Autodesk Inventor part; units mm, degrees
(part 2 of 2)
  spline S114 degree 2 poles (-84.0515, 70.7348) (-84.2812, 70.7348) (-84.6789, 70.8583) (-84.8098, 70.9275) knots 0 0 0 1 2 2 2
  line L120 (-84.8098, 70.9275) -> (-84.8098, 71.3597)
  line L121 (-84.8098, 71.3597) -> (-84.79, 71.3597)
  spline S115 degree 2 poles (-84.79, 71.3597) (-84.7406, 71.3202) (-84.6072, 71.2263) (-84.4961, 71.1745) knots 0 0 0 1 2 2 2
  spline S116 degree 2 poles (-84.4961, 71.1745) (-84.3997, 71.1275) (-84.1626, 71.0584) (-84.0367, 71.0584) knots 0 0 0 1 2 2 2
  spline S117 degree 2 poles (-84.0367, 71.0584) (-83.9453, 71.0584) (-83.7353, 71.1004) (-83.6859, 71.1349) knots 0 0 0 1 2 2 2
  spline S118 degree 2 poles (-83.6859, 71.1349) (-83.6143, 71.1819) (-83.5501, 71.2881) (-83.5501, 71.3968) knots 0 0 0 1 2 2 2
  spline S119 degree 2 poles (-83.5501, 71.3968) (-83.5501, 71.5326) (-83.6983, 71.6734) (-83.8885, 71.7203) knots 0 0 0 1 2 2 2
  spline S120 degree 2 poles (-83.8885, 71.7203) (-83.9626, 71.7376) (-84.1997, 71.787) (-84.3009, 71.8142) knots 0 0 0 1 2 2 2
  spline S121 degree 2 poles (-84.3009, 71.8142) (-84.5628, 71.8908) (-84.7999, 72.2069) (-84.7999, 72.4317) knots 0 0 0 1 2 2 2
  spline S122 degree 2 poles (-84.7999, 72.4317) (-84.7999, 72.7429) (-84.3331, 73.1307) (-83.9477, 73.1307) knots 0 0 0 1 2 2 2
  spline S123 degree 2 poles (-83.9477, 73.1307) (-83.7575, 73.1307) (-83.3722, 73.0369) (-83.2413, 72.9652) knots 0 0 0 1 2 2 2
  line L122 (-83.2413, 72.9652) -> (-83.2413, 72.5527)
  line L123 (-83.2413, 72.5527) -> (-83.2611, 72.5527)
  spline S124 degree 2 poles (-83.2611, 72.5527) (-83.4093, 72.6713) (-83.7699, 72.8071) (-83.9551, 72.8071) knots 0 0 0 1 2 2 2
  spline S125 degree 2 poles (-83.9551, 72.8071) (-84.1453, 72.8071) (-84.4072, 72.6466) (-84.4072, 72.486) knots 0 0 0 1 2 2 2
  spline S126 degree 2 poles (-84.4072, 72.486) (-84.4072, 72.3403) (-84.2515, 72.1995) (-84.0786, 72.1551) knots 0 0 0 1 2 2 2
  spline S127 degree 2 poles (-84.0786, 72.1551) (-83.9947, 72.1328) (-83.7822, 72.0884) (-83.6662, 72.0612) knots 0 0 0 1 2 2 2
  spline S128 degree 2 poles (-83.6662, 72.0612) (-83.4142, 71.997) (-83.1573, 71.703) (-83.1573, 71.4486) knots 0 0 0 1 2 2 2
  spline S129 degree 2 poles (-83.1573, 71.4486) (-83.1573, 71.3004) (-83.2734, 71.0386) (-83.387, 70.9423) knots 0 0 0 1 2 2 2
  spline S130 degree 2 poles (-83.387, 70.9423) (-83.5081, 70.841) (-83.8168, 70.7348) (-84.0515, 70.7348) knots 0 0 0 1 2 2 2
  spline S131 degree 2 poles (-82.1076, 70.7447) (-82.4213, 70.7447) (-82.7745, 71.1028) (-82.7745, 71.4906) knots 0 0 0 1 2 2 2
  line L124 (-82.7745, 71.4906) -> (-82.7745, 72.7577)
  line L125 (-82.7745, 72.7577) -> (-83.0338, 72.7577)
  line L126 (-83.0338, 72.7577) -> (-83.0338, 73.0764)
  line L127 (-83.0338, 73.0764) -> (-82.7745, 73.0764)
  line L128 (-82.7745, 73.0764) -> (-82.7745, 73.7334)
  line L129 (-82.7745, 73.7334) -> (-82.3892, 73.7334)
  line L130 (-82.3892, 73.7334) -> (-82.3892, 73.0764)
  line L131 (-82.3892, 73.0764) -> (-81.6803, 73.0764)
  line L132 (-81.6803, 73.0764) -> (-81.6803, 72.7577)
  line L133 (-81.6803, 72.7577) -> (-82.3892, 72.7577)
  line L134 (-82.3892, 72.7577) -> (-82.3892, 71.6685)
  spline S132 degree 2 poles (-82.3892, 71.6685) (-82.3892, 71.4956) (-82.3768, 71.3054) (-82.3348, 71.2239) knots 0 0 0 1 2 2 2
  spline S133 degree 2 poles (-82.3348, 71.2239) (-82.3002, 71.1522) (-82.1446, 71.0806) (-82.0112, 71.0806) knots 0 0 0 1 2 2 2
  spline S134 degree 2 poles (-82.0112, 71.0806) (-81.9174, 71.0806) (-81.742, 71.1374) (-81.7025, 71.1547) knots 0 0 0 1 2 2 2
  line L135 (-81.7025, 71.1547) -> (-81.6803, 71.1547)
  line L136 (-81.6803, 71.1547) -> (-81.6803, 70.8089)
  spline S135 degree 2 poles (-81.6803, 70.8089) (-81.7889, 70.7793) (-82.0112, 70.7447) (-82.1076, 70.7447) knots 0 0 0 1 2 2 2
  line L137 (-79.3461, 70.7891) -> (-79.3461, 73.4765)
  line L138 (-79.3461, 73.4765) -> (-80.3687, 73.4765)
  line L139 (-80.3687, 73.4765) -> (-80.3687, 73.8371)
  line L140 (-80.3687, 73.8371) -> (-77.9184, 73.8371)
  line L141 (-77.9184, 73.8371) -> (-77.9184, 73.4765)
  line L142 (-77.9184, 73.4765) -> (-78.941, 73.4765)
  line L143 (-78.941, 73.4765) -> (-78.941, 70.7891)
  line L144 (-78.941, 70.7891) -> (-79.3461, 70.7891)
  line L145 (-75.8436, 73.0764) -> (-77.0737, 69.9469)
  line L146 (-77.0737, 69.9469) -> (-77.4862, 69.9469)
  line L147 (-77.4862, 69.9469) -> (-77.0762, 70.9003)
  line L148 (-77.0762, 70.9003) -> (-77.9061, 73.0764)
  line L149 (-77.9061, 73.0764) -> (-77.4911, 73.0764)
  line L150 (-77.4911, 73.0764) -> (-76.8662, 71.3819)
  line L151 (-76.8662, 71.3819) -> (-76.2438, 73.0764)
  line L152 (-76.2438, 73.0764) -> (-75.8436, 73.0764)
  spline S136 degree 2 poles (-73.6354, 71.9945) (-73.6354, 71.4215) (-74.1813, 70.7447) (-74.5987, 70.7447) knots 0 0 0 1 2 2 2
  spline S137 degree 2 poles (-74.5987, 70.7447) (-74.7692, 70.7447) (-75.031, 70.8237) (-75.1668, 70.9052) knots 0 0 0 1 2 2 2
  line L153 (-75.1668, 70.9052) -> (-75.1668, 69.9469)
  line L154 (-75.1668, 69.9469) -> (-75.5522, 69.9469)
  line L155 (-75.5522, 69.9469) -> (-75.5522, 73.0764)
  line L156 (-75.5522, 73.0764) -> (-75.1668, 73.0764)
  line L157 (-75.1668, 73.0764) -> (-75.1668, 72.8368)
  spline S138 degree 2 poles (-75.1668, 72.8368) (-75.0236, 72.9677) (-74.6728, 73.1406) (-74.4678, 73.1406) knots 0 0 0 1 2 2 2
  spline S139 degree 2 poles (-74.4678, 73.1406) (-74.0751, 73.1406) (-73.6354, 72.5181) (-73.6354, 71.9945) knots 0 0 0 1 2 2 2
  spline S140 degree 2 poles (-74.0331, 71.95) (-74.0331, 72.3428) (-74.2826, 72.775) (-74.5617, 72.775) knots 0 0 0 1 2 2 2
  spline S141 degree 2 poles (-74.5617, 72.775) (-74.7247, 72.775) (-75.031, 72.6293) (-75.1668, 72.5157) knots 0 0 0 1 2 2 2
  line L158 (-75.1668, 72.5157) -> (-75.1668, 71.2165)
  spline S142 degree 2 poles (-75.1668, 71.2165) (-75.0162, 71.1448) (-74.8013, 71.0905) (-74.6629, 71.0905) knots 0 0 0 1 2 2 2
  spline S143 degree 2 poles (-74.6629, 71.0905) (-74.3641, 71.0905) (-74.0331, 71.5301) (-74.0331, 71.95) knots 0 0 0 1 2 2 2
  spline S144 degree 2 poles (-72.2423, 70.7373) (-72.7907, 70.7373) (-73.3934, 71.3523) (-73.3934, 71.9204) knots 0 0 0 1 2 2 2
  spline S145 degree 2 poles (-73.3934, 71.9204) (-73.3934, 72.4786) (-72.808, 73.1406) (-72.3362, 73.1406) knots 0 0 0 1 2 2 2
  spline S146 degree 2 poles (-72.3362, 73.1406) (-72.1238, 73.1406) (-71.7953, 73.0171) (-71.6742, 72.8862) knots 0 0 0 1 2 2 2
  spline S147 degree 2 poles (-71.6742, 72.8862) (-71.5507, 72.7553) (-71.4198, 72.3774) (-71.4198, 72.1032) knots 0 0 0 1 2 2 2
  line L159 (-71.4198, 72.1032) -> (-71.4198, 71.8932)
  line L160 (-71.4198, 71.8932) -> (-73.0031, 71.8932)
  spline S148 degree 2 poles (-73.0031, 71.8932) (-73.0031, 71.4956) (-72.603, 71.0732) (-72.2473, 71.0732) knots 0 0 0 1 2 2 2
  spline S149 degree 2 poles (-72.2473, 71.0732) (-72.1213, 71.0732) (-71.8768, 71.13) (-71.778, 71.1745) knots 0 0 0 1 2 2 2
  spline S150 degree 2 poles (-71.778, 71.1745) (-71.6742, 71.2239) (-71.531, 71.3103) (-71.484, 71.3498) knots 0 0 0 1 2 2 2
  line L161 (-71.484, 71.3498) -> (-71.4618, 71.3498)
  line L162 (-71.4618, 71.3498) -> (-71.4618, 70.9299)
  spline S151 degree 2 poles (-71.4618, 70.9299) (-71.5285, 70.9028) (-71.731, 70.8237) (-71.8101, 70.8015) knots 0 0 0 1 2 2 2
  spline S152 degree 2 poles (-71.8101, 70.8015) (-71.9212, 70.7694) (-72.104, 70.7373) (-72.2423, 70.7373) knots 0 0 0 1 2 2 2
  spline S153 degree 2 poles (-71.7953, 72.1872) (-71.8002, 72.3428) (-71.8644, 72.57) (-71.9262, 72.6466) knots 0 0 0 1 2 2 2
  spline S154 degree 2 poles (-71.9262, 72.6466) (-71.9929, 72.733) (-72.2028, 72.8244) (-72.3584, 72.8244) knots 0 0 0 1 2 2 2
  spline S155 degree 2 poles (-72.3584, 72.8244) (-72.5116, 72.8244) (-72.7265, 72.733) (-72.8154, 72.6441) knots 0 0 0 1 2 2 2
  spline S156 degree 2 poles (-72.8154, 72.6441) (-72.9018, 72.5527) (-72.9907, 72.3329) (-73.0031, 72.1872) knots 0 0 0 1 2 2 2
  line L163 (-73.0031, 72.1872) -> (-71.7953, 72.1872)
  point P0 (0, 0)
  constraints: 14 end point, 4 horizontal, 3 collinear, 2 coincident, 2 parallel, 1 perpendicular, 1 point on line, 4 other
extrude "Words" cut sketch "Sketch6" against normal blind 1.27
sketch "Sketch7" plane through (0, 0, 5.08) normal (0, 0, 1) x (1, 0, 0)
  line L0 (94.475, 24.6687) -> (94.475, 8.6687) projected
  line L1 (94.475, 8.6687) -> (76.975, 8.6687) projected
  line L2 (76.975, 8.6687) -> (76.975, 24.6687) projected
  line L3 (76.975, 24.6687) -> (94.475, 24.6687) projected
  line L4 (38.875, 15.8125) -> (38.875, 31.8125) projected
  line L5 (38.875, 31.8125) -> (56.375, 31.8125) projected
  line L6 (56.375, 31.8125) -> (56.375, 15.8125) projected
  line L7 (56.375, 15.8125) -> (38.875, 15.8125) projected
  line L8 (18.275, 17.525) -> (18.275, 1.525) projected
  line L9 (18.275, 1.525) -> (0.775, 1.525) projected
  line L10 (0.775, 1.525) -> (0.775, 17.525) projected
  line L11 (0.775, 17.525) -> (18.275, 17.525) projected
  line L12 (19.825, 11.05) -> (19.825, 27.05) projected
  line L13 (19.825, 27.05) -> (37.325, 27.05) projected
  line L14 (37.325, 27.05) -> (37.325, 11.05) projected
  line L15 (37.325, 11.05) -> (19.825, 11.05) projected
  line L16 (57.925, 11.05) -> (57.925, 27.05) projected
  line L17 (57.925, 27.05) -> (75.425, 27.05) projected
  line L18 (75.425, 27.05) -> (75.425, 11.05) projected
  line L19 (75.425, 11.05) -> (57.925, 11.05) projected
  line L20 (19.825, 30.1) -> (19.825, 46.1) projected
  line L21 (19.825, 46.1) -> (37.325, 46.1) projected
  line L22 (37.325, 46.1) -> (37.325, 30.1) projected
  line L23 (37.325, 30.1) -> (19.825, 30.1) projected
  line L24 (38.875, 34.8625) -> (38.875, 50.8625) projected
  line L25 (38.875, 50.8625) -> (56.375, 50.8625) projected
  line L26 (56.375, 50.8625) -> (56.375, 34.8625) projected
  line L27 (56.375, 34.8625) -> (38.875, 34.8625) projected
  line L28 (18.275, 36.575) -> (18.275, 20.575) projected
  line L29 (18.275, 20.575) -> (0.775, 20.575) projected
  line L30 (0.775, 20.575) -> (0.775, 36.575) projected
  line L31 (0.775, 36.575) -> (18.275, 36.575) projected
  line L32 (57.925, 30.1) -> (57.925, 46.1) projected
  line L33 (57.925, 46.1) -> (75.425, 46.1) projected
  line L34 (75.425, 46.1) -> (75.425, 30.1) projected
  line L35 (75.425, 30.1) -> (57.925, 30.1) projected
  line L36 (94.475, 43.7187) -> (94.475, 27.7187) projected
  line L37 (94.475, 27.7187) -> (76.975, 27.7187) projected
  line L38 (76.975, 27.7187) -> (76.975, 43.7187) projected
  line L39 (76.975, 43.7187) -> (94.475, 43.7187) projected
  line L40 (19.825, 49.15) -> (19.825, 65.15) projected
  line L41 (19.825, 65.15) -> (37.325, 65.15) projected
  line L42 (37.325, 65.15) -> (37.325, 49.15) projected
  line L43 (37.325, 49.15) -> (19.825, 49.15) projected
  line L44 (38.875, 53.9125) -> (38.875, 69.9125) projected
  line L45 (38.875, 69.9125) -> (56.375, 69.9125) projected
  line L46 (56.375, 69.9125) -> (56.375, 53.9125) projected
  line L47 (56.375, 53.9125) -> (38.875, 53.9125) projected
  line L48 (18.275, 55.625) -> (18.275, 39.625) projected
  line L49 (18.275, 39.625) -> (0.775, 39.625) projected
  line L50 (0.775, 39.625) -> (0.775, 55.625) projected
  line L51 (0.775, 55.625) -> (18.275, 55.625) projected
  line L52 (57.925, 49.15) -> (57.925, 65.15) projected
  line L53 (57.925, 65.15) -> (75.425, 65.15) projected
  line L54 (75.425, 65.15) -> (75.425, 49.15) projected
  line L55 (75.425, 49.15) -> (57.925, 49.15) projected
  line L56 (94.475, 62.7687) -> (94.475, 46.7687) projected
  line L57 (94.475, 46.7687) -> (76.975, 46.7687) projected
  line L58 (76.975, 46.7687) -> (76.975, 62.7687) projected
  line L59 (76.975, 62.7687) -> (94.475, 62.7687) projected
  line L60 (99.2197, -0.303) -> (93.9609, -15.4141) projected
  line L61 (93.9609, -15.4141) -> (77.4332, -9.6624) projected
  line L62 (77.4332, -9.6624) -> (82.6919, 5.4488) projected
  line L63 (82.6919, 5.4488) -> (99.2197, -0.303) projected
  line L64 (133.7188, -34.9602) -> (120.2148, -43.5419) projected
  line L65 (120.2148, -43.5419) -> (110.8287, -28.7719) projected
  line L66 (110.8287, -28.7719) -> (124.3326, -20.1903) projected
  line L67 (124.3326, -20.1903) -> (133.7188, -34.9602) projected
  line L68 (50.6581, 5.4488) -> (55.9168, -9.6624) projected
  line L69 (55.9168, -9.6624) -> (39.3891, -15.4141) projected
  line L70 (39.3891, -15.4141) -> (34.1303, -0.303) projected
  line L71 (34.1303, -0.303) -> (50.6581, 5.4488) projected
  line L72 (75.425, 6.6771) -> (75.425, -9.3229) projected
  line L73 (75.425, -9.3229) -> (57.925, -9.3229) projected
  line L74 (57.925, -9.3229) -> (57.925, 6.6771) projected
  line L75 (57.925, 6.6771) -> (75.425, 6.6771) projected
  line L76 (119.3983, -14.7159) -> (109.4651, -27.2591) projected
  line L77 (109.4651, -27.2591) -> (95.746, -16.3947) projected
  line L78 (95.746, -16.3947) -> (105.6792, -3.8515) projected
  line L79 (105.6792, -3.8515) -> (119.3983, -14.7159) projected
  arc A0 (3.175, 74.6125) -> (-3.175, 68.2625) centre (3.175, 68.2625) ccw projected
  line L80 (-3.175, 68.2625) -> (-3.175, 2.8419) projected
  arc A1 (-3.175, 2.8419) -> (2.5106, -3.4733) centre (3.175, 2.8419) ccw projected
  arc A2 (34.1031, -17.9791) -> (2.5106, -3.4733) centre (-3.175, -57.512) ccw projected
  arc A3 (34.1031, -17.9791) -> (41.1537, -19.1093) centre (38.4596, -13.3592) ccw projected
  arc A4 (117.6443, -47.6938) -> (41.1537, -19.1093) centre (65.4005, -70.8608) ccw projected
  arc A5 (120.639, -50.814) -> (139.8041, -35.7732) centre (126.6171, -38.7007) ccw projected
  arc A6 (139.8041, -35.7732) -> (102.6987, 5.8497) centre (84.0124, -48.1591) ccw projected
  arc A7 (98.425, 11.8507) -> (102.6987, 5.8497) centre (104.775, 11.8507) ccw projected
  line L81 (98.425, 11.8507) -> (98.425, 68.2625) projected
  arc A8 (98.425, 68.2625) -> (92.075, 74.6125) centre (92.075, 68.2625) ccw projected
  line L82 (92.075, 74.6125) -> (3.175, 74.6125) projected
  circle A9 centre (3.175, 68.2625) radius 3.81
  circle A10 centre (92.075, 68.2625) radius 3.81
  circle A11 centre (130.4145, -44.6763) radius 3.81
  circle A12 centre (25.7947, -4.4632) radius 3.81
  line L83 (38.875, 69.9125) -> (37.325, 69.9125) construction
  line L84 (37.325, 69.9125) -> (37.325, 65.15) construction
  line L85 (37.325, 65.15) -> (38.875, 65.15) construction
  line L86 (38.875, 65.15) -> (38.875, 69.9125) construction
  line L87 (56.375, 69.9125) -> (57.925, 69.9125) construction
  line L88 (57.925, 69.9125) -> (57.925, 65.15) construction
  line L89 (57.925, 65.15) -> (56.375, 65.15) construction
  line L90 (56.375, 65.15) -> (56.375, 69.9125) construction
  line L91 (57.925, 69.9125) -> (65.5624, 69.9125) construction
  line L92 (65.5624, 69.9125) -> (65.5624, 71.2114) construction
  line L93 (65.5624, 71.2114) -> (57.925, 71.2114) construction
  line L94 (57.925, 71.2114) -> (57.925, 69.9125) construction
  line L95 (65.5624, 69.9125) -> (47.625, 69.9125) construction
  line L96 (47.625, 69.9125) -> (47.625, 80.8323) construction
  line L97 (47.625, 80.8323) -> (65.5624, 80.8323) construction
  line L98 (65.5624, 80.8323) -> (65.5624, 69.9125) construction
  line L99 (37.325, 69.9125) -> (29.6876, 69.9125) construction
  line L100 (29.6876, 69.9125) -> (29.6876, 65.708) construction
  line L101 (29.6876, 65.708) -> (37.325, 65.708) construction
  line L102 (37.325, 65.708) -> (37.325, 69.9125) construction
  line L103 (29.6876, 65.708) -> (47.625, 65.708) construction
  line L104 (47.625, 65.708) -> (47.625, 80.8323) construction
  line L105 (47.625, 80.8323) -> (29.6876, 80.8323) construction
  line L106 (29.6876, 80.8323) -> (29.6876, 65.708) construction
  line L107 (19.825, 65.15) -> (19.825, 84.3808) construction
  line L108 (75.425, 65.15) -> (75.425, 85.1837) construction
  line L109 (130.4145, -44.6763) -> (133.7188, -34.9602) construction
  line L110 (130.4145, -44.6763) -> (120.2148, -43.5419) construction
  circle A13 centre (127.6689, -40.3558) radius 1.309 construction
  circle A14 centre (133.1601, -48.9967) radius 1.309 construction
  line L111 (140.0471, -59.8341) -> (124.0468, -34.6562) construction
  line L112 (133.7188, -34.9602) -> (120.2148, -43.5419) construction
  arc A15 (118.3666, -49.3965) -> (139.8041, -35.7732) centre (126.6171, -38.7007) ccw construction
  circle A16 centre (29.1504, -10.2754) radius 2.9014 construction
  circle A17 centre (32.5061, -4.4632) radius 2.9014 construction
  line L113 (39.3891, -15.4141) -> (34.1303, -0.303) construction
  line L114 (29.1504, -10.2754) -> (25.7947, -4.4632) construction
  line L115 (25.7947, -4.4632) -> (32.5061, -4.4632) construction
  line L116 (32.5061, -4.4632) -> (29.1504, -10.2754) construction
  circle A18 centre (20.5446, -0.2824) radius 2.9014 construction
  line L117 (15.2139, 3.9626) -> (27.0579, -5.4691) construction
  circle A19 centre (25.7947, -4.4632) radius 2.2578
  circle A20 centre (130.4145, -44.6763) radius 2.2578
  circle A21 centre (92.075, 68.2625) radius 2.2578
  circle A22 centre (3.175, 68.2625) radius 2.2578
  arc A23 (117.6443, -47.6938) -> (120.639, -50.814) centre (123.4492, -45.1197) ccw projected
  point P0 (0, 0)
  dimension "d41" = 7.62
  dimension "d42" = 4.5156
  constraints: 66 end point, 12 centre point, 12 parallel, 8 equal radius, 8 tangent, 7 horizontal, 7 perpendicular, 6 coincident, 6 point on line, 4 equal length, 2 vertical, 5 other
  measures "d41" diameter of A9
  measures "d42" diameter of A22
extrude "Extrusion7" cut sketch "Sketch7" against normal blind 25.4 contours A19 | A20 | A21 | A22
sketch "Sketch8" plane through (0, 0, 5.08) normal (0, 0, 1) x (1, 0, 0)
  arc A0 (34.1031, -17.9791) -> (2.5106, -3.4733) centre (-3.175, -57.512) ccw projected
  arc A1 (-3.175, 2.8419) -> (2.5106, -3.4733) centre (3.175, 2.8419) ccw projected
  line L0 (-3.175, 68.2625) -> (-3.175, 2.8419) projected
  arc A2 (3.175, 74.6125) -> (-3.175, 68.2625) centre (3.175, 68.2625) ccw projected
  line L1 (92.075, 74.6125) -> (3.175, 74.6125) projected
  arc A3 (98.425, 68.2625) -> (92.075, 74.6125) centre (92.075, 68.2625) ccw projected
  line L2 (98.425, 11.8507) -> (98.425, 68.2625) projected
  arc A4 (98.425, 11.8507) -> (102.6987, 5.8497) centre (104.775, 11.8507) ccw projected
  arc A5 (139.8041, -35.7732) -> (102.6987, 5.8497) centre (84.0124, -48.1591) ccw projected
  arc A6 (120.639, -50.814) -> (139.8041, -35.7732) centre (126.6171, -38.7007) ccw projected
  arc A7 (117.6443, -47.6938) -> (41.1537, -19.1093) centre (65.4005, -70.8608) ccw construction
  arc A8 (34.1031, -17.9791) -> (41.1537, -19.1093) centre (38.4596, -13.3592) ccw projected
  arc A9 (117.6443, -47.6938) -> (120.639, -50.814) centre (123.4492, -45.1197) ccw projected
  circle A10 centre (104.775, 54.7688) radius 6.35
  circle A11 centre (140.9319, -20.009) radius 6.35
  circle A12 centre (-9.525, 28.575) radius 6.35
  arc A13 (129.1738, -13.1366) -> (137.5618, -14.6271) centre (134.1917, -9.2452) ccw
  line L3 (123.9208, -22.5255) -> (140.9319, -20.009) construction
  line L4 (140.9319, -20.009) -> (131.4297, -34.3414) construction
  arc A14 (139.8041, -35.7732) -> (102.6987, 5.8497) centre (84.0124, -48.1591) ccw projected
  arc A15 (143.1636, -25.9539) -> (139.257, -33.5248) centre (145.3953, -31.8988) ccw
  line L5 (92.725, 61.1688) -> (104.775, 54.7688) construction
  line L6 (104.775, 54.7688) -> (92.725, 48.3688) construction
  arc A16 (98.425, 67.4688) -> (104.775, 61.1188) centre (104.775, 67.4688) ccw
  line L7 (98.425, 11.8507) -> (98.425, 68.2625) construction
  arc A17 (104.775, 48.4188) -> (98.425, 42.0688) centre (104.775, 42.0688) ccw
  line L8 (-9.525, 28.575) -> (2.525, 54.025) construction
  line L9 (-9.525, 28.575) -> (2.525, 3.125) construction
  arc A18 (-9.525, 34.925) -> (-3.175, 41.275) centre (-9.525, 41.275) ccw
  arc A19 (-3.175, 15.875) -> (-9.525, 22.225) centre (-9.525, 15.875) ccw
  circle A20 centre (-9.525, 28.575) radius 2.7027
  circle A21 centre (104.775, 54.7688) radius 2.7027
  circle A22 centre (140.9319, -20.009) radius 2.7027
  line L10 (98.425, 67.4688) -> (98.425, 42.0688)
  point P0 (0, 0)
  dimension "d45" = 12.7
  dimension "d46" = 5.4054
  constraints: 21 point on circle, 15 tangent, 14 end point, 12 centre point, 10 equal radius, 4 point on line, 3 coincident, 3 equal length, 1 collinear
  measures "d45" diameter of A12
  measures "d46" diameter of A20
extrude "Extrusion8" add sketch "Sketch8" against normal up to surface (5.08 mm away)
thread "Thread1" size "1/4-20 UNC" class "2B" standard "ANSI Unified Screw Threads" full length
thread "Thread2" size "1/4-20 UNC" class "2B" standard "ANSI Unified Screw Threads" full length
thread "Thread3" size "1/4-20 UNC" class "2B" standard "ANSI Unified Screw Threads" full length
body "Solid1"
